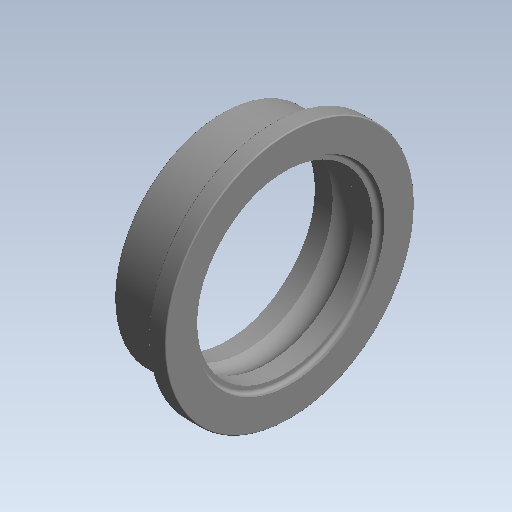
# Autodesk Inventor part: W 619/8 R-2Z_PART2
Saved by Autodesk Inventor 2020 (Build 240168000, 168)
## iProperties
Part Number: W 619/8 R-2Z_PART2
Material: Generic
Catalog Web Link: www.cadenas.de
Description: -Deep groove ball bearings
Vendor: SKF
Document SubType Name: Modeling
Designer: partserver
Manufacturer: SKF
Mass: 0.666807 g
Surface Area: 10.3889 cm^2
Volume: 0.666807 cm^3
Density: 1 g/cm^3
Appearance: PSOLRGB-175-175-175
Category: PARTsolutions
Company: SKF
PSOL_IDENT_0: {$CADENAS_DATA\23d-libs\skf\bearings_units_and_housings\ball_bearings\deep_groove_ball_bearings\bb1_
PSOL_IDENT_1: 001_101.prj},203 {VTYP=3D},{NB=W 619/8 R-2Z_PART2},{LINA=W 619/8 R-2Z_PART2},{NN=BB1_001_101_PART2},
PSOL_IDENT_2: {NOPRJ=TRUE},{DATE=23.12.2020 11:57:27},{GEOMDATE=21.12.2020 15:18:31},{VERSION=},{LINEID=22940},{WB
PSOL_IDENT_3: VAR=},{WBNUMERIC=}  {NB=W 619/8 R-2Z_PART2},{LINA=W 619/8 R-2Z_PART2},{KT=DUMMY},{DESIGNATION=W 619/
PSOL_IDENT_4: 8 R-2Z},{R12=0.30},{DD=8.000},{D=19.000},{B=6.000},{C=},{CX=},{CXX=1.5},{CA=1.500},{XXVARIANT=Flange
PSOL_IDENT_5: d outer ring},{XXDESIGN=Single row stainless steel},{XXSEALING=Shield on both sides},{DESIGN=dgbbwr2
PSOL_IDENT_6: zs},{DESIGNIR=dgbbwr2zs},{VARIANT=Flanged outer ring},{DD1=10.50},{DD2=9.8},{DD2X=},{DD2A=9.80},{D1=
PSOL_IDENT_7: 15.50},{D1X=MIN},{D2=16.66},{D2A=16.66},{D3=22},{D3X=},{D3A=22.000},{D4=},{HH=MIN},{BB=MIN},{BBX=},{
PSOL_IDENT_8: BBA=0.000},{FF=},{R0MAX=MIN},{R0=MIN},{PITCH=13.00},{DW=3.175},{DDAMIN=9.700},{DDAMAX=9.700},{DDBMIN=
PSOL_IDENT_9: MIN},{DDBMAX=MIN},{DBMIN=MIN},{DAMAX=MIN},{BBAMIN=MIN},{CAMAX=MIN},{RAMAX=0.300},{LOAD1=1.250},{LOAD
PSOL_IDENT_10: 2=0.455},{LOAD3=0.020},{SPEED1=85000},{SPEED2=43000},{KR=0.025},{F0=6.600},{Z=7},{II=1},{MASS=0.008}
PSOL_IDENT_11: ,{BEARING=W 619/8 R-2Z},{RING=},{HELP=1.750},{HELP2=1.170},{DD1ALG=5.250},{YALG=5.250},{PITCH1=13.00
PSOL_IDENT_12: 0},{DW1=3.175},{YALG1=7.750},{HALG1=1.750},{SH=4.900},{CU=0.565},{HALG=1.25},{B1=-3.22875},{SHIELDHE
PSOL_IDENT_13: LP=2},{D4A=0.000},{FFA=0.000},{RS1=}
NB: W 619/8 R-2Z_PART2
NT: Deep groove ball bearings
NBSYN: $DESIGNATION._PART2
LINA: W 619/8 R-2Z_PART2
CATALOG: SKF
SUPPLIER: SKF
ARTICLENO: W 619/8 R-2Z_PART2
BOMINFO: W 619/8 R-2Z_PART2
CREATOR: CADENAS GmbH
Title: W 619/8 R-2Z_PART2
Author: Cadenas PARTsolutions
Comments: Deep groove ball bearings
Autodesk Inventor part; units mm, degrees
ref_plane "YZ Plane" through (0, 0, 0) normal (1, 0, 0) x (0, 1, 0)
ref_plane "XZ Plane" through (0, 0, 0) normal (0, 1, 0) x (-1, 0, 0)
ref_plane "XY Plane" through (0, 0, 0) normal (0, 0, 1) x (1, 0, 0)
sketch "Sketch_21" plane through (0, 0, 0) normal (0, 0, 1) x (1, 0, 0)
  line L0 (50, 0) -> (-50, 0)
  line L1 (0, 10.9) -> (0, 8.33)
  line L2 (0, 8.33) -> (0.15, 8.33)
  arc A0 (0.45, 8.03) -> (0.15, 8.33) centre (0.15, 8.03) ccw
  line L3 (0.45, 8.03) -> (0.45, 7.75)
  line L4 (0.45, 7.75) -> (2.0214, 7.75)
  arc A1 (3.9786, 7.75) -> (2.0214, 7.75) centre (3, 6.5) ccw
  line L5 (3.9786, 7.75) -> (5.55, 7.75)
  line L6 (5.55, 7.75) -> (5.55, 8.03)
  arc A2 (5.85, 8.33) -> (5.55, 8.03) centre (5.85, 8.03) ccw
  line L7 (5.85, 8.33) -> (6, 8.33)
  line L8 (6, 8.33) -> (6, 9.4)
  arc A3 (6, 9.4) -> (5.9, 9.5) centre (5.9, 9.4) ccw
  line L9 (5.9, 9.5) -> (1.5, 9.5)
  line L10 (1.5, 9.5) -> (1.5, 10.9)
  arc A4 (1.5, 10.9) -> (1.4, 11) centre (1.4, 10.9) ccw
  line L11 (1.4, 11) -> (0.1, 11)
  arc A5 (0.1, 11) -> (0, 10.9) centre (0.1, 10.9) ccw
  constraints: 24 end point, 12 point on circle, 6 centre point
revolve "Revolution1" add sketch "Sketch_21" angle 360 about axis through (50, 0, 0) along (1, 0, 0)
body "Solid1"
